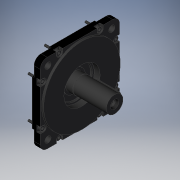
# Autodesk Inventor part: AKM2G-5ACDNCA_F
Saved by Autodesk Inventor 2019 (Build 230136000, 136)
## iProperties
Created: 2024-01-27
Part Number: AKM2G-5ACDNCA_F
Material: Generic
Catalog Web Link: www.cadenas.de
Description: AKM2G Size 5 - Front-AKM2G Series
Vendor: KOLLMORGEN
Document SubType Name: Modeling
Designer: psAdmin
Manufacturer: KOLLMORGEN
Mass: 171.637 g
Surface Area: 416.965 cm^2
Volume: 171.637 cm^3
Density: 1 g/cm^3
Appearance: PSOLRGB-175-175-175
Category: PARTsolutions
Company: KOLLMORGEN
Title: AKM2G-5ACDNCA_F
Author: Cadenas PARTsolutions
Comments: AKM2G Series
PSOL_IDENT_0: {$CADENAS_DATA/23d-libs/kollmorgen/akm2g/parts/akm2g5_front.prj},199 {VTYP=3D},{NB=AKM2G-5ACDNCA_F},
PSOL_IDENT_1: {LINA=AKM2G-5ACDNCA_F},{NN=AKM2G Size 5 - Front},{DATE=28.07.2023 05:36:25},{GEOMDATE=28.07.2023 05:
PSOL_IDENT_2: 24:00},{VERSION=},{LINEID=10},{WBVAR=MO,SH,CON,BR,FD},{WBNUMERIC=}  {NB=AKM2G-5ACDNCA_F},{LINA=AKM2G
PSOL_IDENT_3: -5ACDNCA_F},{KT=DUMMY},{PN=AKM2G-5ACDNCA},{FS=Size 5},{MO=A},{SH=C},{CON=D},{BR=N},{FD=CA},{FDALG='C
PSOL_IDENT_4: A','Sfd3 smart feedback','GF','Multi-turn hiperface dsl','LD','Multi-turn inductive endat 2.2'},{B=2
PSOL_IDENT_5: .5}
NB: AKM2G-5ACDNCA_F
NN: AKM2G Size 5 - Front
NT: AKM2G Series
NBSYN: $PN._F
LINA: AKM2G-5ACDNCA_F
CATALOG: Kollmorgen
FS: Size 5
MO: A = Metric IEC
SH: Closed keyway
CON: Single right angle M23
BR: No brake
FD: Sfd3 smart feedback
SUPPLIER: KOLLMORGEN
ARTICLENO: AKM2G-5ACDNCA_F
BOMINFO: AKM2G-5ACDNCA_F
CREATOR: CADENAS GmbH
Autodesk Inventor part; units mm, degrees
ref_plane "YZ Plane" through (0, 0, 0) normal (1, 0, 0) x (0, 1, 0)
ref_plane "XZ Plane" through (0, 0, 0) normal (0, 1, 0) x (-1, 0, 0)
ref_plane "XY Plane" through (0, 0, 0) normal (0, 0, 1) x (1, 0, 0)
sketch "Sketch_1" plane through (0, 0, 0) normal (1, 0, 0) x (0, 1, 0)
  arc A0 (-47, 57) -> (-57, 47) centre (-47, 47) ccw
  line L0 (-57, 47) -> (-57, -47)
  arc A1 (-57, -47) -> (-47, -57) centre (-47, -47) ccw
  line L1 (-47, -57) -> (47, -57)
  arc A2 (47, -57) -> (57, -47) centre (47, -47) ccw
  line L2 (57, -47) -> (57, 47)
  arc A3 (57, 47) -> (47, 57) centre (47, 47) ccw
  line L3 (47, 57) -> (-47, 57)
  constraints: 8 end point, 8 point on circle, 4 centre point
extrude "Extrusion1" add sketch "Sketch_1" along normal blind 9
sketch "Sketch_2" plane through (0, 0, 0) normal (1, 0, 0) x (0, 1, 0)
  line L0 (-32.5, 57) -> (-32.5, 43.5)
  arc A0 (-43.5, 32.5) -> (-32.5, 43.5) centre (-43.5, 43.5) ccw
  line L1 (-43.5, 32.5) -> (-57, 32.5)
  line L2 (-57, 32.5) -> (-57, -32.5)
  line L3 (-57, -32.5) -> (-43.5, -32.5)
  arc A1 (-32.5, -43.5) -> (-43.5, -32.5) centre (-43.5, -43.5) ccw
  line L4 (-32.5, -43.5) -> (-32.5, -57)
  line L5 (-32.5, -57) -> (32.5, -57)
  line L6 (32.5, -57) -> (32.5, -43.5)
  arc A2 (43.5, -32.5) -> (32.5, -43.5) centre (43.5, -43.5) ccw
  line L7 (43.5, -32.5) -> (57, -32.5)
  line L8 (57, -32.5) -> (57, 32.5)
  line L9 (57, 32.5) -> (43.5, 32.5)
  arc A3 (32.5, 43.5) -> (43.5, 32.5) centre (43.5, 43.5) ccw
  line L10 (32.5, 43.5) -> (32.5, 57)
  line L11 (32.5, 57) -> (-32.5, 57)
  constraints: 24 end point, 8 point on circle, 4 centre point
extrude "Extrusion2" add sketch "Sketch_2" against normal blind 2.5
sketch "Sketch_3" plane through (0, 0, 0) normal (0, 0, 1) x (1, 0, 0)
  line L0 (12, 0) -> (9, 0)
  line L1 (9, 0) -> (9, 55)
  line L2 (9, 55) -> (12, 55)
  line L3 (12, 55) -> (12, 0)
  line L4 (12, 0) -> (9, 0)
  constraints: 10 end point
revolve "Revolution1" add sketch "Sketch_3" angle 360 about axis through (12, 0, 0) along (1, 0, 0)
sketch "Sketch_4" plane through (0, 0, 0) normal (0, 0, 1) x (1, 0, 0)
  line L0 (12, 0) -> (3.5, 0)
  line L1 (0.5, 23.5) -> (0.5, 15.9)
  line L2 (0.5, 15.9) -> (1, 15.9)
  line L3 (1, 15.9) -> (1, 12.5)
  line L4 (1, 12.5) -> (11, 12.5)
  line L5 (11, 12.5) -> (11, 12)
  line L6 (11, 12) -> (12, 12)
  line L7 (12, 12) -> (12, 26)
  line L8 (12, 26) -> (3.5, 26)
  line L9 (3.5, 26) -> (3.5, 23.5)
  line L10 (3.5, 23.5) -> (0.5, 23.5)
  constraints: 22 end point
revolve "Revolution2" cut sketch "Sketch_4" angle 360 about axis through (12, 0, 0) along (1, 0, 0)
sketch "Sketch_5" plane through (0, 0, 0) normal (0, 0, 1) x (1, 0, 0)
  line L0 (59, 0) -> (12, 0)
  line L1 (12, 0) -> (12, 12)
  line L2 (12, 12) -> (59, 12)
  line L3 (59, 12) -> (59, 0)
  line L4 (59, 0) -> (12, 0)
  constraints: 10 end point
revolve "Revolution3" add sketch "Sketch_5" angle 360 about axis through (59, 0, 0) along (1, 0, 0)
sketch "Sketch6" plane through (0, 0, 0) normal (-1, 0, 0) x (0, 0, 1)
  point P0 (-45.9619, 45.9619)
hole "Hole1" at (0, 45.9619, -45.9619) direction (1, 0, 0) diameter 9 depth 9
sketch "Sketch7" plane through (0, 0, 0) normal (-1, 0, 0) x (0, 0, 1)
  point P0 (-45.9619, -45.9619)
hole "Hole2" at (0, -45.9619, -45.9619) direction (1, 0, 0) diameter 9 depth 9
sketch "Sketch8" plane through (0, 0, 0) normal (-1, 0, 0) x (0, 0, 1)
  point P0 (45.9619, 45.9619)
hole "Hole3" at (0, 45.9619, 45.9619) direction (1, 0, 0) diameter 9 depth 9
sketch "Sketch9" plane through (0, 0, 0) normal (-1, 0, 0) x (0, 0, 1)
  point P0 (45.9619, -45.9619)
hole "Hole4" at (0, -45.9619, 45.9619) direction (1, 0, 0) diameter 9 depth 9
sketch "Sketch_11" plane through (9, 0, 0) normal (1, 0, 0) x (0, 0, -1)
  line L0 (-116.6139, 92.3035) -> (-116.6139, -93.0632)
  line L1 (-116.6139, -93.0632) -> (124.2109, -93.0632)
  line L2 (124.2109, -93.0632) -> (124.2109, 92.3035)
  line L3 (124.2109, 92.3035) -> (-116.6139, 92.3035)
  line L4 (-57, -33.635) -> (-57, -57)
  line L5 (-57, -57) -> (-33.63, -57)
  line L6 (-33.63, -57) -> (-33.63, -52.7)
  arc A0 (-24.78, -52.7) -> (-33.63, -52.7) centre (-29.205, -52.7) ccw
  line L7 (-24.78, -52.7) -> (-24.78, -57)
  line L8 (-24.78, -57) -> (24.78, -57)
  line L9 (24.78, -57) -> (24.78, -52.7)
  arc A1 (33.63, -52.7) -> (24.78, -52.7) centre (29.205, -52.7) ccw
  line L10 (33.63, -52.7) -> (33.63, -57)
  line L11 (33.63, -57) -> (57, -57)
  line L12 (57, -57) -> (57, -33.635)
  line L13 (57, -33.635) -> (52.7, -33.635)
  arc A2 (52.7, -24.785) -> (52.7, -33.635) centre (52.7, -29.21) ccw
  line L14 (52.7, -24.785) -> (57, -24.785)
  line L15 (57, -24.785) -> (57, 24.785)
  line L16 (57, 24.785) -> (52.7, 24.785)
  arc A3 (52.7, 33.635) -> (52.7, 24.785) centre (52.7, 29.21) ccw
  line L17 (52.7, 33.635) -> (57, 33.635)
  line L18 (57, 33.635) -> (57, 57)
  line L19 (57, 57) -> (33.63, 57)
  line L20 (33.63, 57) -> (33.63, 52.7)
  arc A4 (24.78, 52.7) -> (33.63, 52.7) centre (29.205, 52.7) ccw
  line L21 (24.78, 52.7) -> (24.78, 57)
  line L22 (24.78, 57) -> (-24.78, 57)
  line L23 (-24.78, 57) -> (-24.78, 52.7)
  arc A5 (-33.63, 52.7) -> (-24.78, 52.7) centre (-29.205, 52.7) ccw
  line L24 (-33.63, 52.7) -> (-33.63, 57)
  line L25 (-33.63, 57) -> (-57, 57)
  line L26 (-57, 57) -> (-57, 33.635)
  line L27 (-57, 33.635) -> (-52.7, 33.635)
  arc A6 (-52.7, 24.785) -> (-52.7, 33.635) centre (-52.7, 29.21) ccw
  line L28 (-52.7, 24.785) -> (-57, 24.785)
  line L29 (-57, 24.785) -> (-57, -24.785)
  line L30 (-57, -24.785) -> (-52.7, -24.785)
  arc A7 (-52.7, -33.635) -> (-52.7, -24.785) centre (-52.7, -29.21) ccw
  line L31 (-52.7, -33.635) -> (-57, -33.635)
  constraints: 64 end point, 16 point on circle, 8 centre point
extrude "Extrusion3" cut sketch "Sketch_11" against normal blind 5
sketch "Sketch_17" plane through (0, 0, -15) normal (0, 0, 1) x (1, 0, 0)
  arc A0 (14, 0) -> (18, -4) centre (18, 0) ccw
  line L0 (18, -4) -> (50, -4)
  arc A1 (50, -4) -> (54, 0) centre (50, 0) ccw
  arc A2 (54, 0) -> (50, 4) centre (50, 0) ccw
  line L1 (50, 4) -> (18, 4)
  arc A3 (18, 4) -> (14, 0) centre (18, 0) ccw
  constraints: 8 point on circle, 4 centre point, 4 end point
extrude "Extrusion4" add sketch "Sketch_17" along normal blind 4
sketch "Sketch_6" plane through (0, 0, 0) normal (0, 0, 1) x (1, 0, 0)
  line L0 (59, 0) -> (32.037, 0)
  line L1 (32.037, 0) -> (34, 3.4)
  line L2 (34, 3.4) -> (52.2, 3.4)
  line L3 (52.2, 3.4) -> (53, 4.2)
  line L4 (53, 4.2) -> (55.71, 4.2)
  line L5 (55.71, 4.2) -> (59, 6.1)
  line L6 (59, 6.1) -> (59, 0)
  line L7 (59, 0) -> (32.037, 0)
  constraints: 16 end point
revolve "Revolution4" cut sketch "Sketch_6" angle 360 about axis through (59, 0, 0) along (1, 0, 0)
sketch "Sketch_12" plane through (0, 0, -29.21) normal (0, 0, 1) x (1, 0, 0)
  line L0 (-12, 52.7) -> (8, 52.7)
  line L1 (8, 52.7) -> (8, 49.4475)
  line L2 (8, 49.4475) -> (7.7525, 49.2)
  line L3 (7.7525, 49.2) -> (4.2475, 49.2)
  line L4 (4.2475, 49.2) -> (4, 49.4475)
  line L5 (4, 49.4475) -> (4, 51.2)
  line L6 (4, 51.2) -> (-11.7525, 51.2)
  line L7 (-11.7525, 51.2) -> (-12, 51.4475)
  line L8 (-12, 51.4475) -> (-12, 52.7)
  line L9 (-12, 52.7) -> (8, 52.7)
  constraints: 20 end point
revolve "Revolution5" add sketch "Sketch_12" angle 360 about axis through (-12, 52.7, -29.21) along (-1, 0, 0)
sketch "Pattern_1_SKETCH_1" plane through (0, 0, 29.21) normal (0, 0, 1) x (1, 0, 0)
  line L0 (-12, 52.7) -> (8, 52.7)
  line L1 (8, 52.7) -> (8, 49.4475)
  line L2 (8, 49.4475) -> (7.7525, 49.2)
  line L3 (7.7525, 49.2) -> (4.2475, 49.2)
  line L4 (4.2475, 49.2) -> (4, 49.4475)
  line L5 (4, 49.4475) -> (4, 51.2)
  line L6 (4, 51.2) -> (-11.7525, 51.2)
  line L7 (-11.7525, 51.2) -> (-12, 51.4475)
  line L8 (-12, 51.4475) -> (-12, 52.7)
  line L9 (-12, 52.7) -> (8, 52.7)
  constraints: 20 end point
sketch "Pattern_1_SKETCH_2" plane through (0, -23.49, 52.7) normal (0, 0, 1) x (1, 0, 0)
  line L0 (-12, 52.7) -> (8, 52.7)
  line L1 (8, 52.7) -> (8, 49.4475)
  line L2 (8, 49.4475) -> (7.7525, 49.2)
  line L3 (7.7525, 49.2) -> (4.2475, 49.2)
  line L4 (4.2475, 49.2) -> (4, 49.4475)
  line L5 (4, 49.4475) -> (4, 51.2)
  line L6 (4, 51.2) -> (-11.7525, 51.2)
  line L7 (-11.7525, 51.2) -> (-12, 51.4475)
  line L8 (-12, 51.4475) -> (-12, 52.7)
  line L9 (-12, 52.7) -> (8, 52.7)
  constraints: 20 end point
sketch "Pattern_1_SKETCH_3" plane through (0, -23.49, -52.7) normal (0, 0, 1) x (1, 0, 0)
  line L0 (-12, 52.7) -> (8, 52.7)
  line L1 (8, 52.7) -> (8, 49.4475)
  line L2 (8, 49.4475) -> (7.7525, 49.2)
  line L3 (7.7525, 49.2) -> (4.2475, 49.2)
  line L4 (4.2475, 49.2) -> (4, 49.4475)
  line L5 (4, 49.4475) -> (4, 51.2)
  line L6 (4, 51.2) -> (-11.7525, 51.2)
  line L7 (-11.7525, 51.2) -> (-12, 51.4475)
  line L8 (-12, 51.4475) -> (-12, 52.7)
  line L9 (-12, 52.7) -> (8, 52.7)
  constraints: 20 end point
sketch "Pattern_1_SKETCH_4" plane through (0, 0, 29.21) normal (0, 0, 1) x (1, 0, 0)
  line L0 (-12, -52.7) -> (8, -52.7)
  line L1 (8, -52.7) -> (8, -55.9525)
  line L2 (8, -55.9525) -> (7.7525, -56.2)
  line L3 (7.7525, -56.2) -> (4.2475, -56.2)
  line L4 (4.2475, -56.2) -> (4, -55.9525)
  line L5 (4, -55.9525) -> (4, -54.2)
  line L6 (4, -54.2) -> (-11.7525, -54.2)
  line L7 (-11.7525, -54.2) -> (-12, -53.9525)
  line L8 (-12, -53.9525) -> (-12, -52.7)
  line L9 (-12, -52.7) -> (8, -52.7)
  constraints: 20 end point
sketch "Pattern_1_SKETCH_5" plane through (0, 0, -29.21) normal (0, 0, 1) x (1, 0, 0)
  line L0 (-12, -52.7) -> (8, -52.7)
  line L1 (8, -52.7) -> (8, -55.9525)
  line L2 (8, -55.9525) -> (7.7525, -56.2)
  line L3 (7.7525, -56.2) -> (4.2475, -56.2)
  line L4 (4.2475, -56.2) -> (4, -55.9525)
  line L5 (4, -55.9525) -> (4, -54.2)
  line L6 (4, -54.2) -> (-11.7525, -54.2)
  line L7 (-11.7525, -54.2) -> (-12, -53.9525)
  line L8 (-12, -53.9525) -> (-12, -52.7)
  line L9 (-12, -52.7) -> (8, -52.7)
  constraints: 20 end point
sketch "Pattern_1_SKETCH_6" plane through (0, -23.49, 52.7) normal (0, 0, 1) x (1, 0, 0)
  line L0 (-12, -5.72) -> (8, -5.72)
  line L1 (8, -5.72) -> (8, -8.9725)
  line L2 (8, -8.9725) -> (7.7525, -9.22)
  line L3 (7.7525, -9.22) -> (4.2475, -9.22)
  line L4 (4.2475, -9.22) -> (4, -8.9725)
  line L5 (4, -8.9725) -> (4, -7.22)
  line L6 (4, -7.22) -> (-11.7525, -7.22)
  line L7 (-11.7525, -7.22) -> (-12, -6.9725)
  line L8 (-12, -6.9725) -> (-12, -5.72)
  line L9 (-12, -5.72) -> (8, -5.72)
  constraints: 20 end point
sketch "Pattern_1_SKETCH_7" plane through (0, -23.49, -52.7) normal (0, 0, 1) x (1, 0, 0)
  line L0 (-12, -5.72) -> (8, -5.72)
  line L1 (8, -5.72) -> (8, -8.9725)
  line L2 (8, -8.9725) -> (7.7525, -9.22)
  line L3 (7.7525, -9.22) -> (4.2475, -9.22)
  line L4 (4.2475, -9.22) -> (4, -8.9725)
  line L5 (4, -8.9725) -> (4, -7.22)
  line L6 (4, -7.22) -> (-11.7525, -7.22)
  line L7 (-11.7525, -7.22) -> (-12, -6.9725)
  line L8 (-12, -6.9725) -> (-12, -5.72)
  line L9 (-12, -5.72) -> (8, -5.72)
  constraints: 20 end point
revolve "Revolution6" add sketch "Pattern_1_SKETCH_1" angle 360 about axis through (-12, 52.7, 29.21) along (-1, 0, 0)
revolve "Revolution7" add sketch "Pattern_1_SKETCH_2" angle 360 about axis through (-12, 29.21, 52.7) along (-1, 0, 0)
revolve "Revolution8" add sketch "Pattern_1_SKETCH_3" angle 360 about axis through (-12, 29.21, -52.7) along (-1, 0, 0)
revolve "Revolution9" add sketch "Pattern_1_SKETCH_4" angle 360 about axis through (-12, -52.7, 29.21) along (-1, 0, 0)
revolve "Revolution10" add sketch "Pattern_1_SKETCH_5" angle 360 about axis through (-12, -52.7, -29.21) along (-1, 0, 0)
revolve "Revolution11" add sketch "Pattern_1_SKETCH_6" angle 360 about axis through (-12, -29.21, 52.7) along (-1, 0, 0)
revolve "Revolution12" add sketch "Pattern_1_SKETCH_7" angle 360 about axis through (-12, -29.21, -52.7) along (-1, 0, 0)
sketch "Sketch_26" plane through (8, 0, 0) normal (1, 0, 0) x (0, 0, -1)
  line L0 (27.705, 51.834) -> (29.205, 50.9679)
  line L1 (29.205, 50.9679) -> (30.705, 51.834)
  line L2 (30.705, 51.834) -> (30.705, 53.566)
  line L3 (30.705, 53.566) -> (29.205, 54.4321)
  line L4 (29.205, 54.4321) -> (27.705, 53.566)
  line L5 (27.705, 53.566) -> (27.705, 51.834)
  constraints: 12 end point
extrude "Extrusion5" cut sketch "Sketch_26" along normal mid plane 4
sketch "Pattern_3_SKETCH_1" plane through (8, 0, 0) normal (1, 0, 0) x (0, 0, -1)
  line L0 (-30.71, 51.834) -> (-29.21, 50.9679)
  line L1 (-29.21, 50.9679) -> (-27.71, 51.834)
  line L2 (-27.71, 51.834) -> (-27.71, 53.566)
  line L3 (-27.71, 53.566) -> (-29.21, 54.4321)
  line L4 (-29.21, 54.4321) -> (-30.71, 53.566)
  line L5 (-30.71, 53.566) -> (-30.71, 51.834)
  constraints: 12 end point
sketch "Pattern_3_SKETCH_2" plane through (8, 0, 0) normal (1, 0, 0) x (0, 0, -1)
  line L0 (-54.2, 28.344) -> (-52.7, 27.4779)
  line L1 (-52.7, 27.4779) -> (-51.2, 28.344)
  line L2 (-51.2, 28.344) -> (-51.2, 30.076)
  line L3 (-51.2, 30.076) -> (-52.7, 30.9421)
  line L4 (-52.7, 30.9421) -> (-54.2, 30.076)
  line L5 (-54.2, 30.076) -> (-54.2, 28.344)
  constraints: 12 end point
sketch "Pattern_3_SKETCH_3" plane through (8, 0, 0) normal (1, 0, 0) x (0, 0, -1)
  line L0 (51.2, 28.344) -> (52.7, 27.4779)
  line L1 (52.7, 27.4779) -> (54.2, 28.344)
  line L2 (54.2, 28.344) -> (54.2, 30.076)
  line L3 (54.2, 30.076) -> (52.7, 30.9421)
  line L4 (52.7, 30.9421) -> (51.2, 30.076)
  line L5 (51.2, 30.076) -> (51.2, 28.344)
  constraints: 12 end point
sketch "Pattern_3_SKETCH_4" plane through (8, 0, 0) normal (1, 0, 0) x (0, 0, -1)
  line L0 (-30.71, -53.566) -> (-29.21, -54.4321)
  line L1 (-29.21, -54.4321) -> (-27.71, -53.566)
  line L2 (-27.71, -53.566) -> (-27.71, -51.834)
  line L3 (-27.71, -51.834) -> (-29.21, -50.9679)
  line L4 (-29.21, -50.9679) -> (-30.71, -51.834)
  line L5 (-30.71, -51.834) -> (-30.71, -53.566)
  constraints: 12 end point
sketch "Pattern_3_SKETCH_5" plane through (8, 0, 0) normal (1, 0, 0) x (0, 0, -1)
  line L0 (27.71, -53.566) -> (29.21, -54.4321)
  line L1 (29.21, -54.4321) -> (30.71, -53.566)
  line L2 (30.71, -53.566) -> (30.71, -51.834)
  line L3 (30.71, -51.834) -> (29.21, -50.9679)
  line L4 (29.21, -50.9679) -> (27.71, -51.834)
  line L5 (27.71, -51.834) -> (27.71, -53.566)
  constraints: 12 end point
sketch "Pattern_3_SKETCH_6" plane through (8, 0, 0) normal (1, 0, 0) x (0, 0, -1)
  line L0 (-54.2, -30.076) -> (-52.7, -30.9421)
  line L1 (-52.7, -30.9421) -> (-51.2, -30.076)
  line L2 (-51.2, -30.076) -> (-51.2, -28.344)
  line L3 (-51.2, -28.344) -> (-52.7, -27.4779)
  line L4 (-52.7, -27.4779) -> (-54.2, -28.344)
  line L5 (-54.2, -28.344) -> (-54.2, -30.076)
  constraints: 12 end point
sketch "Pattern_3_SKETCH_7" plane through (8, 0, 0) normal (1, 0, 0) x (0, 0, -1)
  line L0 (51.2, -30.076) -> (52.7, -30.9421)
  line L1 (52.7, -30.9421) -> (54.2, -30.076)
  line L2 (54.2, -30.076) -> (54.2, -28.344)
  line L3 (54.2, -28.344) -> (52.7, -27.4779)
  line L4 (52.7, -27.4779) -> (51.2, -28.344)
  line L5 (51.2, -28.344) -> (51.2, -30.076)
  constraints: 12 end point
extrude "Extrusion6" cut sketch "Pattern_3_SKETCH_1" along normal mid plane 4
extrude "Extrusion7" cut sketch "Pattern_3_SKETCH_2" along normal mid plane 4
extrude "Extrusion8" cut sketch "Pattern_3_SKETCH_3" along normal mid plane 4
extrude "Extrusion9" cut sketch "Pattern_3_SKETCH_4" along normal mid plane 4
extrude "Extrusion10" cut sketch "Pattern_3_SKETCH_5" along normal mid plane 4
extrude "Extrusion11" cut sketch "Pattern_3_SKETCH_6" along normal mid plane 4
extrude "Extrusion12" cut sketch "Pattern_3_SKETCH_7" along normal mid plane 4
ref_plane "F_XY" through (-2.5, 0, 0) normal (1, 0, 0) x (0, 0, -1)
ref_plane "F_YZ" through (-2.5, 0, 0) normal (0, 0, -1) x (0, 1, 0)
ref_plane "F_ZX" through (-2.5, 0, 0) normal (0, 1, 0) x (1, 0, 0)
ref_plane "SH_SEAL_XY" through (9, 0, 0) normal (1, 0, 0) x (0, 0, -1)
ref_plane "SH_SEAL_YZ" through (9, 0, 0) normal (0, 0, -1) x (0, 1, 0)
ref_plane "SH_SEAL_ZX" through (9, 0, 0) normal (0, 1, 0) x (1, 0, 0)
body "Solid1"
